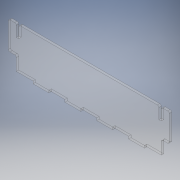
# Autodesk Inventor part: back_v2
Saved by Autodesk Inventor 2017.2 (Build 212233000, 233)
## iProperties
Created: 2017-06-09
Part Number: back_v2
Material: Generic
Document SubType Name: Modeling
Designer: SandeepSH
Density: 1 g/cm^3
Appearance: Polycarbonate - Clear
Author: SandeepSH
Autodesk Inventor part; units mm, degrees
ref_plane "YZ Plane" through (0, 0, 0) normal (1, 0, 0) x (0, 1, 0)
ref_plane "XZ Plane" through (0, 0, 0) normal (0, 1, 0) x (-1, 0, 0)
ref_plane "XY Plane" through (0, 0, 0) normal (0, 0, 1) x (1, 0, 0)
sketch "Sketch1" plane through (0, 0, 0) normal (0, 0, 1) x (1, 0, 0)
  line L0 (0, 0) -> (182, 0)
  line L1 (182, 0) -> (182, 55)
  line L2 (182, 55) -> (0, 55)
  line L3 (0, 55) -> (0, 0)
  dimension "d0" = 182
  dimension "d1" = 55
  constraints: 8 end point, 2 parallel, 1 horizontal, 1 perpendicular
  measures "d0" distance of L2.end L1.end
  measures "d1" distance of L1.end L0.end
extrude "Extrusion1" add sketch "Sketch1" along normal blind 3
sketch "Sketch2" plane through (0, 0, 3) normal (0, 0, 1) x (1, 0, 0)
  line L0 (0, 0) -> (21, 0)
  line L1 (21, 0) -> (21, 3)
  line L2 (21, 3) -> (0, 3)
  line L3 (0, 3) -> (0, 0)
  line L4 (0, 0) -> (182, 0) projected
  line L5 (41, 0) -> (61, 0)
  line L6 (61, 0) -> (61, 3)
  line L7 (61, 3) -> (41, 3)
  line L8 (41, 3) -> (41, 0)
  line L9 (81, 0) -> (101, 0)
  line L10 (101, 0) -> (101, 3)
  line L11 (101, 3) -> (81, 3)
  line L12 (81, 3) -> (81, 0)
  line L13 (121, 0) -> (141, 0)
  line L14 (141, 0) -> (141, 3)
  line L15 (141, 3) -> (121, 3)
  line L16 (121, 3) -> (121, 0)
  line L17 (182, 0) -> (161, 0)
  line L18 (161, 0) -> (161, 3)
  line L19 (161, 3) -> (182, 3)
  line L20 (182, 3) -> (182, 0)
  dimension "d4" = 21
  dimension "d5" = 3
  dimension "d6" = 20
  dimension "d7" = 3
  dimension "d8" = 20
  dimension "d9" = 20
  dimension "d10" = 3
  dimension "d11" = 20
  dimension "d12" = 20
  dimension "d13" = 3
  dimension "d14" = 20
  dimension "d35" = 21
  dimension "d36" = 3
  dimension "d37" = 20
  constraints: 40 end point, 10 parallel, 5 horizontal, 5 perpendicular, 3 point on line
  measures "d4" distance of L2.end L1.end
  measures "d5" distance of L1.end L0.end
  measures "d6" distance of L7.end L6.end
  measures "d7" distance of L6.end L5.end
  measures "d8" distance between parallel lines of L8 L1
  measures "d9" distance of L11.end L10.end
  measures "d10" distance of L10.end L9.end
  measures "d11" distance from line of L11.end L6
  measures "d12" distance of L15.end L14.end
  measures "d13" distance of L14.end L13.end
  measures "d14" distance between parallel lines of L16 L10
  measures "d35" distance of L18.end L19.end
  measures "d36" distance of L17.end L18.end
  measures "d37" distance between parallel lines of L18 L14
sketch "Sketch3" plane through (0, 0, 3) normal (0, 0, 1) x (1, 0, 0)
  line L0 (182, 55) -> (0, 55) projected
  line L1 (0, 55) -> (3, 55)
  line L2 (3, 55) -> (3, 40)
  line L3 (3, 40) -> (0, 40)
  line L4 (0, 40) -> (0, 55)
  line L5 (182, 55) -> (179, 55)
  line L6 (179, 55) -> (179, 40)
  line L7 (179, 40) -> (182, 40)
  line L8 (182, 40) -> (182, 55)
  point P0 (0, 0)
  dimension "d22" = 3
  dimension "d23" = 15
  dimension "d24" = 3
  dimension "d25" = 15
  constraints: 16 end point, 4 parallel, 2 horizontal, 2 perpendicular
  measures "d22" distance of L2.end L3.end
  measures "d23" distance of L1.end L2.end
  measures "d24" distance of L7.end L6.end
  measures "d25" distance of L6.end L5.end
extrude "Extrusion3" cut sketch "Sketch3" against normal through all
sketch "Sketch4" plane through (0, 0, 3) normal (0, 0, 1) x (1, 0, 0)
  line L0 (179, 55) -> (3, 55) projected
  line L1 (0, 55) -> (-10, 55)
  line L2 (-10, 55) -> (-10, 20)
  line L3 (-10, 20) -> (0, 20)
  line L4 (0, 20) -> (0, 55)
  line L5 (0, 0) -> (182, 0) projected
  line L6 (182, 0) -> (182, 40) projected
  line L7 (182, 55) -> (192, 55)
  line L8 (192, 55) -> (192, 20)
  line L9 (192, 20) -> (182, 20)
  line L10 (182, 20) -> (182, 55)
  line L11 (0, 0) -> (182, 0) projected
  line L12 (0, 40) -> (0, 0) projected
  point P0 (25, 0)
  point P1 (45, 0)
  point P2 (172, 3)
  point P3 (182, 40)
  point P4 (185, 0)
  point P5 (205, 0)
  dimension "d28" = 10
  dimension "d29" = 20
  dimension "d30" = 10
  dimension "d31" = 20
  constraints: 16 end point, 4 parallel, 3 collinear, 2 horizontal, 2 perpendicular, 1 vertical, 1 other
  measures "d28" distance of L3.end L2.end
  measures "d29" distance between parallel lines of L5 L3
  measures "d30" distance of L8.end L9.end
  measures "d31" distance between parallel lines of L11 L9
extrude "Extrusion4" add sketch "Sketch4" against normal blind 3
fillet "Fillet1" radius 2 10 edges at (3, 55, 1.5) (0, 55, 1.5) (-10, 55, 1.5) (-10, 20, 1.5) (0, 20, 1.5) (192, 20, 1.5) (182, 20, 1.5) (192, 55, 1.5) (179, 55, 1.5) (182, 55, 1.5) curvature continuous yes
extrude "Extrusion5" cut sketch "Sketch2" against normal through all
equation "\"d11\" = d6"
equation "\"d14\" = d11"
equation "\"d35\" = d4"
body "Solid1"
